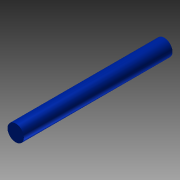
# Autodesk Inventor part: MU_Prolene_Offset
Saved by Autodesk Inventor 2011 SP2 (Build 150309200, 309)
## iProperties
Created: 2011-01-13
Part Number: MU_Prolene_Offset
Document SubType Name: Modeling
Designer: sungwook
Density: 0.91 g/cm^3
Material: PP
Mass: 0.000421947 g
Surface Area: 0.0510765 cm^2
Volume: 0.000463678 cm^3
Author: sungwook
Autodesk Inventor part; units mm, degrees
ref_plane "YZ Plane" through (0, 0, 0) normal (1, 0, 0) x (0, 1, 0)
ref_plane "XZ Plane" through (0, 0, 0) normal (0, 1, 0) x (-1, 0, 0)
ref_plane "XY Plane" through (0, 0, 0) normal (0, 0, 1) x (1, 0, 0)
sketch "Sketch1" plane through (0, 0, 0) normal (0, 0, 1) x (1, 0, 0)
  circle A0 centre (0, 0) radius 0.19
  dimension "d0" = 0.38
  constraints: 1 centre point, 1 coincident
  measures "d0" diameter of A0
extrude "Extrusion1" add sketch "Sketch1" along normal blind 3.45
equation "\"d0\" = dFlexure"
equation "\"d1\" = offset_fl_adj"
equation "\"baseInitD\" = 4"
equation "\"baseTh0\" = 48.463041deg"
equation "\"baseTh1\" = 23.073918deg"
equation "\"topD\" = 14"
equation "\"topInitD\" = 4"
equation "\"topTh0\" = 16.60155deg"
equation "\"topTh1\" = 86.796901deg"
equation "\"lFlexure\" = 1.5"
equation "\"dFlexure\" = 0.38"
equation "\"springBaseD\" = 8"
equation "\"springTopD\" = 8"
equation "\"dMotor\" = 1.44"
equation "\"springInitL\" = 12.7"
equation "\"lMotor\" = 22.35"
equation "\"topH\" = 21.66629"
equation "\"springL\" = 30.86629"
equation "\"springLset\" = 3.5"
equation "\"springDeform\" = 18.16629"
equation "\"springUnderCut\" = 9.2"
equation "\"spirngLO\" = 31.67176"
equation "\"springLO\" = 33.86629"
equation "\"lFlexureOffset\" = 1.95"
equation "\"dM1X\" = 6.73587"
equation "\"dM2X\" = -1.34133"
equation "\"dM1Y\" = 2.34012"
equation "\"dM2Y\" = 7.00349"
equation "\"dM1Xt\" = 6.59227"
equation "\"dM1Yt\" = -0.43704"
equation "\"dM2Yt\" = 5.49055"
equation "\"dM2Xt\" = -3.67462"
equation "\"GuideRod\" = 2"
equation "\"baseOD\" = 23"
equation "\"GuideTubingID\" = 2"
equation "\"CSpringCD\" = 0.254"
equation "\"CSpringOD\" = 5.537"
equation "\"GuideTubingOD\" = 4"
equation "\"CSpringID\" = 5.029"
equation "\"offset_fl_adj\" = lFlexure + lFlexureOffset"
equation "\"OCToffset\" = 14.38"
equation "\"lOCTprobe\" = 75"
equation "\"lOCT\" = 58"
equation "\"lOCTprobeNorm\" = 72.38"
equation "\"lOCTprobeNom\" = 72.38"
body "Solid1"
